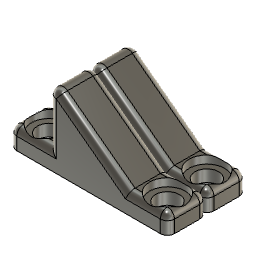
_paper guide mount.fa4ce9f8-fc40-4f42-b492-7d3dc72e7cbd (Autodesk Fusion 360 design; units mm, degrees)
Autodesk Fusion 360 part; units mm, degrees
note: some values were not read from the file. Set by a fixed rule: which sketch regions a step uses.
sketch "Sketch1" plane through (0, 0, 0) normal (0, 0, 1) x (1, 0, 0)
  line L0 (0, 0) -> (-20, 0)
  line L1 (-20, 0) -> (-20, 10)
  line L2 (-20, 10) -> (0, 10)
  line L3 (0, 10) -> (0, 0)
  dimension "d1" = 20
  dimension "d2" = 10
  constraint horizontal L0
  constraint vertical L1
  constraint horizontal L2
  constraint vertical L3
  constraint coincident L0.start L3.end
  measures "d1" distance of L0.start L0.end
  measures "d2" distance of L0.start L2.end
extrude "Extrude1" add sketch "Sketch1" along normal blind 20 makes body 1
sketch "Sketch2" plane through (0, 0, 0) normal (0, -1, 0) x (1, 0, 0)
  line L0 (-20, 0) -> (0, 0)
  line L1 (0, 0) -> (0, 20)
  line L2 (0, 20) -> (-20, 20)
  line L3 (-20, 20) -> (-20, 0)
  circle A0 centre (-10, 8) radius 7.5
  line L4 (-10, 8) -> (-12, 10)
  line L5 (-12, 10) -> (-13.4142, 8.5858)
  line L6 (-13.4142, 8.5858) -> (-11.4142, 6.5858)
  line L7 (-11.4142, 6.5858) -> (-10, 8)
  circle A1 centre (-11.4142, 6.5858) radius 7.5
  line L8 (-15.9631, 12.5488) -> (-5.4512, 12.5488)
  line L9 (-5.4512, 12.5488) -> (-5.4512, 2.0369)
  line L10 (-5.4512, 2.0369) -> (-15.9631, 2.0369)
  line L11 (-15.9631, 2.0369) -> (-15.9631, 12.5488)
  line L12 (-15.9631, 12.5488) -> (-5.4512, 2.0369) construction
  line L13 (-5.4512, 12.5488) -> (-15.9631, 2.0369) construction
  line L14 (-15.9631, 12.5488) -> (-5.4512, 2.0369)
  line L15 (-5.4512, 2.0369) -> (-5.5395, 1.9486)
  line L16 (-5.5395, 1.9486) -> (-16.0514, 12.4605)
  line L17 (-16.0514, 12.4605) -> (-15.9631, 12.5488)
  point P0 (-10.7071, 7.2929)
  dimension "d5" = 15
  dimension "d6" = 2
  dimension "d7" = 15
  dimension "d8" = 0.125
  constraint perpendicular L4 L5
  constraint parallel L4 L6
  constraint parallel L5 L7
  constraint coincident A0.centre L4.start
  constraint coincident L6.end L7.start
  constraint horizontal L8
  constraint perpendicular L8 L9
  constraint parallel L8 L10
  constraint parallel L9 L11
  constraint coincident L12 P0
  constraint coincident L13 P0
  constraint coincident A1 L8.start
  constraint coincident A0 L8.start
  constraint midpoint L7 P0
  constraint perpendicular L14 L15
  constraint parallel L14 L16
  constraint parallel L15 L17
  measures "d5" diameter of A0
  measures "d6" distance of A0.centre L6.end
  measures "d7" diameter of A1
  measures "d8" distance of L8.start L16.end
extrude "Extrude2" cut sketch "Sketch2" against normal blind 5 contours A0 L11 L16 | A0 L5 L6 L7 L10 L11 L16 | A0 L10 L16 | L5 L6 L7 L16 picked at (-16.1588, 6.7234) picked at (-11.2766, 1.8412) bodies 1
sketch "Sketch3" plane through (0, 0, 0) normal (1, 0, 0) x (0, 1, 0)
  line L0 (0, 0) -> (10, 0)
  line L1 (10, 0) -> (10, 5)
  line L2 (10, 5) -> (0, 5)
  line L3 (0, 5) -> (0, 0)
  dimension "d13" = 10
  dimension "d14" = 5
  constraint horizontal L0
  constraint vertical L1
  constraint horizontal L2
  constraint vertical L3
  constraint coincident L0.start L3.end
  measures "d13" distance of L0.start L0.end
  measures "d14" distance of L0.start L2.end
extrude "Extrude3" add sketch "Sketch3" along normal blind 10 bodies 1
sketch "Sketch4" plane through (-20, 0, 0) normal (-1, 0, 0) x (0, -1, 0)
  line L0 (-10, 0) -> (0, 0)
  line L1 (0, 0) -> (0, 20)
  line L2 (0, 20) -> (-10, 20)
  line L3 (-10, 20) -> (-10, 0)
  line L4 (-10, 0) -> (0, 0)
  line L5 (0, 0) -> (0, 5)
  line L6 (0, 5) -> (-10, 5)
  line L7 (-10, 5) -> (-10, 0)
  dimension "d17" = 10
  dimension "d18" = 5
  constraint horizontal L4
  constraint vertical L5
  constraint horizontal L6
  constraint vertical L7
  constraint coincident L0.start L3.end
  measures "d17" distance of L0.start L0.end
  measures "d18" distance of L0.start L6.end
extrude "Extrude4" add sketch "Sketch4" along normal blind 10 contours L0 L1 L3 L4 L5 L6 L7 bodies 1
sketch "Sketch5" plane through (0, 0, 5) normal (0, 0, 1) x (-1, 0, 0)
  line L0 (0, -10) -> (0, 0)
  line L1 (0, 0) -> (-10, 0)
  line L2 (-10, 0) -> (-10, -10)
  line L3 (-10, -10) -> (0, -10)
  circle A0 centre (-5, -5) radius 3
  circle A1 centre (25, -5) radius 3
  dimension "d21" = 6
  dimension "d22" = 6
  measures "d21" diameter of A0
  measures "d22" diameter of A1
extrude "Extrude5" cut sketch "Sketch5" against normal blind 5 contours A0 | A1 bodies 1
sketch "Sketch6" plane through (0, 0, 5) normal (0, 0, 1) x (-1, 0, 0)
  circle A0 centre (-5, -5) radius 3
  line L0 (0, -10) -> (0, 0)
  line L1 (0, 0) -> (-10, 0)
  line L2 (-10, 0) -> (-10, -10)
  line L3 (-10, -10) -> (0, -10)
  circle A1 centre (25, -5) radius 4.5
  circle A2 centre (-5, -5) radius 4.5
  dimension "d25" = 9
  dimension "d26" = 9
  constraint concentric A0 A2
  measures "d25" diameter of A1
  measures "d26" diameter of A2
extrude "Extrude6" cut sketch "Sketch6" against normal blind 2 contours A1 | A2 bodies 1
sketch "Sketch7" plane through (0, 0, 0) normal (0, -1, 0) x (1, 0, 0)
  line L0 (-16.0388, 12.4478) -> (-5.5522, 1.9612)
  arc A0 (-16.0388, 12.4478) -> (-5.5522, 1.9612) centre (-10, 8) ccw
  line L1 (0, 5) -> (0, 20)
  line L2 (0, 20) -> (-20, 20)
  line L3 (-30, 0) -> (10, 0)
  line L4 (0, 5) -> (-20, 20)
  line L5 (-20, 20) -> (-10.1377, 33.1497)
  line L6 (-10.1377, 33.1497) -> (9.8623, 18.1497)
  line L7 (9.8623, 18.1497) -> (0, 5)
  line L8 (10, 0) -> (10, 5)
  line L9 (10, 5) -> (0, 5)
  line L10 (-20, 20) -> (-20, 5)
  line L11 (-20, 5) -> (-30, 5)
  line L12 (-30, 5) -> (-30, 0)
  constraint perpendicular L4 L5
  constraint parallel L4 L6
  constraint parallel L5 L7
  constraint coincident L1 L4.start
extrude "Extrude7" cut sketch "Sketch7" against normal blind 10 contours L1 L2 L4 bodies 1
fillet "Fillet2" radius 1.8 15 edges at (-30, 0, 2.5) (-25, 0, 5) (-20, 0, 12.5) (-30, 5, 5) (5, 0, 5) (10, 5, 5) (10, 0, 2.5) (10, 10, 2.5) (5, 10, 5) (-20, 10, 12.5) (-25, 10, 5) (-30, 10, 2.5) (-10, 0, 12.5) (-10, 10, 12.5) (-20, 5, 20) on bodies 1
mirror "Mirror1" about plane through (0, 0, 0) normal (0, 1, 0) of bodies 1 makes body 2
